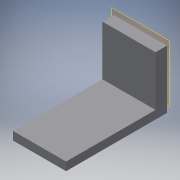
# Autodesk Inventor part: fotel
Saved by Autodesk Inventor 2017 (Build 210142000, 142)
## iProperties
Created: 2016-11-30
Part Number: fotel
Material: Generic
Document SubType Name: Modeling
Designer: Marcin
Mass: 13500 g
Surface Area: 18210.4 cm^2
Volume: 66412.3 cm^3
Density: 0.203275 g/cm^3
Appearance: Default
Author: Marcin
Autodesk Inventor part; units mm, degrees
ref_plane "YZ Plane" through (0, 0, 0) normal (1, 0, 0) x (0, 1, 0)
ref_plane "XZ Plane" through (0, 0, 0) normal (0, 1, 0) x (-1, 0, 0)
ref_plane "XY Plane" through (0, 0, 0) normal (0, 0, 1) x (1, 0, 0)
ref_plane "Work Plane1" through (0, 0, 0) normal (0, 0, 1) x (1, 0, 0)
sketch "Sketch1" plane through (0, 0, 0) normal (0, 0, 1) x (1, 0, 0)
  line L0 (255, -336.4839) -> (-255, -336.4839)
  line L1 (-255, -336.4839) -> (-255, 223.5161)
  line L2 (-255, 223.5161) -> (255, 223.5161)
  line L3 (255, 223.5161) -> (255, -336.4839)
  line L4 (255, -336.4839) -> (-255, 223.5161) construction
  line L5 (-255, -336.4839) -> (255, 223.5161) construction
  point P0 (0, -56.4839)
  dimension "d0" = 510
  dimension "d1" = 560
  constraints: 12 end point, 2 midpoint, 2 parallel, 1 horizontal, 1 perpendicular
  measures "d0" distance of L1.end L2.end
  measures "d1" distance of L0.end L1.end
extrude "Extrusion1" add sketch "Sketch1" along normal blind 110
sketch "Sketch2" plane through (0, 0, 110) normal (0, 0, 1) x (1, 0, 0)
  line L0 (-255, -336.4839) -> (255, -336.4839) projected
  line L1 (255, -336.4839) -> (255, 223.5161) projected
  line L2 (-255, -336.4839) -> (255, -336.4839)
  line L3 (255, -336.4839) -> (255, -256.6929)
  line L4 (255, -256.6929) -> (-255, -256.6929)
  line L5 (-255, -256.6929) -> (-255, -336.4839)
  point P0 (0, 0)
  constraints: 8 end point, 2 parallel, 1 horizontal, 1 perpendicular, 1 point on line
extrude "Extrusion2" add sketch "Sketch2" along normal blind 860
body "Solid1"
